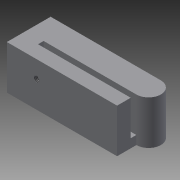
# Autodesk Inventor part: Standard (DIN)
Saved by Autodesk Inventor 2014 (Build 180170000, 170)
## iProperties
Shininess: 64.0
Length Units: 11269
Angle Units: 11279
Time Units: 11290
Mass Units: 11283
Length Display Precision: 3
Angle Display Precision: 2
Compacted: True
Part Number: Standard (DIN)
Document SubType Name: Modeling
Density: 1 g/cm^3
Material: Generisch
Appearance: Vorgabe
Density: 0.0
Volumn: 0.0
Area: 0.0
PropertySet Name: Model Information
Control State: 0
Master: False
Checked Out: False
Autodesk Inventor part; units mm, degrees
ref_plane "YZ Plane" through (0, 0, 0) normal (1, 0, 0) x (0, 1, 0)
ref_plane "XZ Plane" through (0, 0, 0) normal (0, 1, 0) x (-1, 0, 0)
ref_plane "XY Plane" through (0, 0, 0) normal (0, 0, 1) x (1, 0, 0)
sketch "Skizze8" plane through (0, 0, 0) normal (0, 0, 1) x (1, 0, 0)
  line L0 (-31.4655, -12.5) -> (31.4655, -12.5)
  line L1 (31.4655, -12.5) -> (31.4655, 12.5)
  line L2 (31.4655, 12.5) -> (-31.4655, 12.5)
  line L3 (-31.4655, 12.5) -> (-31.4655, -12.5)
  line L4 (-31.4655, -12.5) -> (31.4655, 12.5) construction
  line L5 (31.4655, -12.5) -> (-31.4655, 12.5) construction
  point P0 (0, 0)
  dimension "d28" = 62.931
  dimension "d29" = 25
  constraints: 12 end point, 2 midpoint, 2 parallel, 1 horizontal, 1 perpendicular
  measures "d28" distance of L2.end L1.end
  measures "d29" distance of L1.end L0.end
extrude "Extrusion7" add sketch "Skizze8" along normal blind 5
sketch "Skizze9" plane through (0, 0, 5) normal (0, 0, 1) x (1, 0, 0)
  line L0 (31.4655, 12.5) -> (-31.4655, 12.5) projected
  line L1 (-31.4655, 12.5) -> (-31.4655, -12.5) projected
  line L2 (-31.4655, -12.5) -> (-21.4655, -12.5)
  line L3 (-21.4655, -12.5) -> (-21.4655, 12.5)
  line L4 (-21.4655, 12.5) -> (-31.4655, 12.5)
  line L5 (-31.4655, 12.5) -> (-31.4655, -12.5)
  point P0 (0, 0)
  dimension "d32" = 10
  constraints: 8 end point, 2 parallel, 1 horizontal, 1 perpendicular, 1 point on line
  measures "d32" distance of L4.end L3.end
extrude "Extrusion8" add sketch "Skizze9" along normal blind 20
sketch "Skizze10" plane through (0, 0, 5) normal (0, 0, 1) x (1, 0, 0)
  line L0 (-21.4655, 12.5) -> (38.4655, 12.5)
  line L1 (38.4655, 12.5) -> (38.4655, -1.5)
  line L2 (38.4655, -1.5) -> (-21.4655, -1.5)
  line L3 (-21.4655, -1.5) -> (-21.4655, 12.5)
  point P0 (0, 0)
  dimension "d35" = 59.931
  dimension "d36" = 14
  constraints: 8 end point, 2 parallel, 1 horizontal, 1 perpendicular
  measures "d35" distance of L1.end L2.end
  measures "d36" distance of L0.end L1.end
extrude "Extrusion9" add sketch "Skizze10" along normal blind 20
fillet "Rundung4" radius 7 2 edges at (38.4655, 12.5, 15) (38.4655, -1.5, 15)
sketch "Skizze11" plane through (0, 0, 5) normal (0, 0, 1) x (1, 0, 0)
  line L0 (31.4655, -12.5) -> (31.4655, -1.5) projected
  line L1 (-21.4655, -12.5) -> (31.4655, -12.5)
  line L2 (31.4655, -12.5) -> (31.4655, -4.7)
  line L3 (31.4655, -4.7) -> (-21.4655, -4.7)
  line L4 (-21.4655, -4.7) -> (-21.4655, -12.5)
  point P0 (0, 0)
  dimension "d40" = 7.8
  constraints: 8 end point, 2 parallel, 1 horizontal, 1 perpendicular, 1 point on line
  measures "d40" distance of L2.end L1.end
extrude "Extrusion10" add sketch "Skizze11" along normal blind 20
sketch "Skizze12" plane through (-31.4655, -12.5, 0) normal (0, -1, 0) x (1, 0, 0)
  line L0 (0, 25) -> (62.931, 25) projected
  line L1 (10, 25) -> (10, 5) projected
  point P0 (31.4655, 0)
  point P1 (17, 15.1)
  dimension "d43" = 7
  dimension "d44" = 9.9
  measures "d43" distance from line of L1 point (17, 15.1)
  measures "d44" distance from line of L0 point (17, 15.1)
hole "Bohrung1" at (-14.4655, -12.5, 15.1) direction (0, 1, 0) diameter 3.242 depth 20 tip angle 118 thread size "M4x0.7" class "6H" standard "ANSI Metric M Profile"
sketch "Skizze13" plane through (0, 0, 5) normal (0, 0, -1) x (-1, 0, 0)
  arc A0 (-31.4655, 12.5) -> (-31.4655, -1.5) centre (-31.4655, 5.5) ccw projected
  line L0 (-31.4655, -1.5) -> (-31.4655, 12.5) projected
  line L1 (-31.4655, -12.5) -> (-31.4655, 12.5) projected
  point P0 (0, 0)
extrude "Extrusion11" add sketch "Skizze13" along normal blind 5
